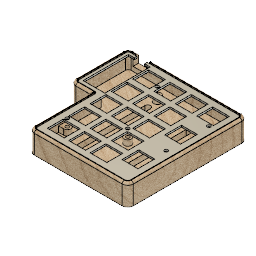
yampad_v3-Fusion360 (Autodesk Fusion 360 design; units mm, degrees)
Autodesk Fusion 360 part; units mm, degrees
note: some values were not read from the file. Set by a fixed rule: which sketch regions a step uses.
(part 1 of 2)
sketch "yampad_v2-Eco2.User-screws" plane through (0, 0, 0) normal (0, 1, 0) x (1, 0, 0) in component "Plate"
  line L0 (16.764, -31.877) -> (-1.397, -31.877) construction
  line L1 (71.501, -52.959) -> (57.531, -52.959) construction
  circle A0 centre (20.066, -74.613) radius 3.2553 construction
  line L2 (76.581, -81.534) -> (76.581, -67.564) construction
  line L3 (38.481, -0.889) -> (52.451, -0.889) construction
  line L4 (57.531, -52.959) -> (57.531, -38.989) construction
  line L5 (52.451, -0.889) -> (52.451, -14.859) construction
  line L6 (90.551, -67.564) -> (90.551, -81.534) construction
  circle A1 centre (54.991, -55.499) radius 3.2528 construction
  line L7 (33.401, -0.889) -> (33.401, -14.859) construction
  line L8 (90.551, -81.534) -> (76.581, -81.534) construction
  line L9 (11.557, -2.286) -> (3.937, -2.286) construction
  line L10 (3.937, 3.048) -> (11.557, 3.048) construction
  line L11 (3.937, -2.286) -> (3.937, 3.048) construction
  line L12 (57.531, -38.989) -> (71.501, -38.989) construction
  line L13 (16.764, 1.524) -> (16.764, -31.877) construction
  line L14 (33.401, -14.859) -> (19.431, -14.859) construction
  line L15 (19.431, -0.889) -> (33.401, -0.889) construction
  line L16 (-1.397, 1.524) -> (16.764, 1.524) construction
  line L17 (19.431, -14.859) -> (19.431, -0.889) construction
  line L18 (76.581, -29.464) -> (90.551, -29.464) construction
  line L19 (11.557, 3.048) -> (11.557, -2.286) construction
  line L20 (90.551, -43.434) -> (76.581, -43.434) construction
  line L21 (71.501, -38.989) -> (71.501, -52.959) construction
  line L22 (-1.397, -31.877) -> (-1.524, 1.524) construction
  line L23 (33.401, -33.909) -> (19.431, -33.909) construction
  line L24 (52.451, -14.859) -> (38.481, -14.859) construction
  line L25 (38.481, -52.959) -> (38.481, -38.989) construction
  line L26 (38.481, -33.909) -> (38.481, -19.939) construction
  line L27 (33.401, -58.039) -> (33.401, -72.009) construction
  line L28 (33.401, -19.939) -> (33.401, -33.909) construction
  line L29 (57.531, -58.039) -> (71.501, -58.039) construction
  line L30 (90.551, -14.859) -> (76.581, -14.859) construction
  line L31 (76.581, -43.434) -> (76.581, -29.464) construction
  line L32 (71.501, -33.909) -> (57.531, -33.909) construction
  line L33 (52.451, -52.959) -> (38.481, -52.959) construction
  line L34 (57.531, -33.909) -> (57.531, -19.939) construction
  line L35 (33.401, -52.959) -> (19.431, -52.959) construction
  line L36 (19.431, -52.959) -> (19.431, -38.989) construction
  line L37 (19.431, -19.939) -> (33.401, -19.939) construction
  line L38 (71.501, -19.939) -> (71.501, -33.909) construction
  line L39 (57.531, -14.859) -> (57.531, -0.889) construction
  line L40 (38.481, -14.859) -> (38.481, -0.889) construction
  circle A2 centre (35.941, -9.906) radius 3.2553 construction
  circle A3 centre (89.408, -17.399) radius 3.2453 construction
  line L41 (38.481, -19.939) -> (52.451, -19.939) construction
  line L42 (57.531, -19.939) -> (71.501, -19.939) construction
  line L43 (57.531, -0.889) -> (71.501, -0.889) construction
  line L44 (71.501, -14.859) -> (57.531, -14.859) construction
  line L45 (76.581, -14.859) -> (76.581, -0.889) construction
  line L46 (52.451, -19.939) -> (52.451, -33.909) construction
  line L47 (33.401, -38.989) -> (33.401, -52.959) construction
  line L48 (76.581, -67.564) -> (90.551, -67.564) construction
  circle A4 centre (89.408, -55.499) radius 3.2379 construction
  line L49 (52.451, -33.909) -> (38.481, -33.909) construction
  line L50 (90.551, -0.889) -> (90.551, -14.859) construction
  line L51 (19.431, -58.039) -> (33.401, -58.039) construction
  line L52 (76.581, -0.889) -> (90.551, -0.889) construction
  line L53 (38.481, -72.009) -> (38.481, -58.039) construction
  line L54 (38.481, -38.989) -> (52.451, -38.989) construction
  line L55 (19.431, -38.989) -> (33.401, -38.989) construction
  line L56 (33.401, -77.089) -> (33.401, -91.059) construction
  line L57 (71.501, -58.039) -> (71.501, -72.009) construction
  line L58 (52.451, -91.059) -> (38.481, -91.059) construction
  line L59 (19.431, -72.009) -> (19.431, -58.039) construction
  line L60 (90.551, -29.464) -> (90.551, -43.434) construction
  line L61 (52.451, -38.989) -> (52.451, -52.959) construction
  line L62 (71.501, -0.889) -> (71.501, -14.859) construction
  line L63 (19.431, -33.909) -> (19.431, -19.939) construction
  line L64 (71.501, -91.059) -> (57.531, -91.059) construction
  line L65 (33.401, -72.009) -> (19.431, -72.009) construction
  line L66 (57.531, -72.009) -> (57.531, -58.039) construction
  line L67 (38.481, -91.059) -> (38.481, -77.089) construction
  line L68 (19.431, -91.059) -> (19.431, -77.089) construction
  line L69 (52.451, -77.089) -> (52.451, -91.059) construction
  line L70 (57.531, -77.089) -> (71.501, -77.089) construction
  line L71 (71.501, -77.089) -> (71.501, -91.059) construction
  line L72 (52.451, -72.009) -> (38.481, -72.009) construction
  line L73 (71.501, -72.009) -> (57.531, -72.009) construction
  line L74 (19.431, -77.089) -> (33.401, -77.089) construction
  line L75 (38.481, -58.039) -> (52.451, -58.039) construction
  line L76 (52.451, -58.039) -> (52.451, -72.009) construction
  line L77 (33.401, -91.059) -> (19.431, -91.059) construction
  line L78 (57.531, -91.059) -> (57.531, -77.089) construction
  line L79 (38.481, -77.089) -> (52.451, -77.089) construction
sketch "yampad_v2-Edge.Cuts" plane through (0, 0, 0) normal (0, 1, 0) x (1, 0, 0) in component "Plate"
  arc A0 (16.51, -91.694) -> (18.288, -93.472) centre (18.288, -91.694) ccw construction
  line L0 (18.288, -93.472) -> (91.44, -93.472) construction
  line L1 (15.24, -38.354) -> (-0.254, -38.354) construction
  arc A1 (-1.524, -37.084) -> (-0.254, -38.354) centre (-0.254, -37.084) ccw construction
  line L2 (-1.524, -37.084) -> (-1.524, 0) construction
  line L3 (91.186, 1.524) -> (0, 1.524) construction
  arc A2 (0, 1.524) -> (-1.524, 0) centre (0, 0) ccw construction
  arc A3 (92.964, -0.254) -> (91.186, 1.524) centre (91.186, -0.254) ccw construction
  line L4 (16.51, -91.694) -> (16.51, -39.624) construction
  arc A4 (16.51, -39.624) -> (15.24, -38.354) centre (15.24, -39.624) ccw construction
  line L5 (92.964, -91.948) -> (92.964, -0.254) construction
  arc A5 (91.44, -93.472) -> (92.964, -91.948) centre (91.44, -91.948) ccw construction
sketch "Sketch3" plane through (0, 0, 0) normal (0, 1, 0) x (1, 0, 0) in component "Plate"
  line L0 (18.288, -93.472) -> (91.44, -93.472) construction
  arc A0 (16.51, -91.694) -> (18.288, -93.472) centre (18.288, -91.694) ccw construction
  line L1 (16.51, -91.694) -> (16.51, -39.624) construction
  arc A1 (16.51, -39.624) -> (15.24, -38.354) centre (15.24, -39.624) ccw construction
  line L2 (15.24, -38.354) -> (-0.254, -38.354) construction
  arc A2 (-1.524, -37.084) -> (-0.254, -38.354) centre (-0.254, -37.084) ccw construction
  line L3 (-1.524, -37.084) -> (-1.524, 0) construction
  arc A3 (0, 1.524) -> (-1.524, 0) centre (0, 0) ccw construction
  line L4 (91.186, 1.524) -> (0, 1.524) construction
  arc A4 (92.964, -0.254) -> (91.186, 1.524) centre (91.186, -0.254) ccw construction
  line L5 (92.964, -91.948) -> (92.964, -0.254) construction
  arc A5 (91.44, -93.472) -> (92.964, -91.948) centre (91.44, -91.948) ccw construction
  line L6 (91.44, -93.472) -> (92.964, -93.472) construction
  line L7 (92.964, -93.472) -> (92.964, -91.948) construction
  line L8 (91.186, 1.524) -> (92.964, 1.524) construction
  line L9 (92.964, 1.524) -> (92.964, -0.254) construction
  line L10 (-1.524, 0) -> (-1.524, 1.524) construction
  line L11 (0, 1.524) -> (-1.524, 1.524) construction
  line L12 (-1.524, -37.084) -> (-1.524, -38.354) construction
  line L13 (-1.524, -38.354) -> (-0.254, -38.354) construction
  line L14 (16.51, -91.694) -> (16.51, -93.472) construction
  line L15 (16.51, -93.472) -> (18.288, -93.472) construction
  line L16 (18.288, -96.472) -> (91.44, -96.472)
  line L17 (91.44, -96.472) -> (93.964, -96.472)
  line L18 (95.964, -94.472) -> (95.964, -91.948)
  line L19 (95.964, -91.948) -> (95.964, -0.254)
  line L20 (95.964, 2.524) -> (95.964, -0.254)
  line L21 (91.186, 4.524) -> (93.964, 4.524)
  line L22 (91.186, 4.524) -> (0, 4.524)
  line L23 (0, 4.524) -> (-2.524, 4.524)
  line L24 (-4.524, 0) -> (-4.524, 2.524)
  line L25 (-4.524, -37.084) -> (-4.524, 0)
  line L26 (-4.524, -37.084) -> (-4.524, -39.354)
  line L27 (-2.524, -41.354) -> (-0.254, -41.354)
  line L28 (11.51, -41.354) -> (-0.254, -41.354)
  line L29 (13.51, -91.694) -> (13.51, -43.354)
  line L30 (13.51, -91.694) -> (13.51, -94.472)
  line L31 (15.51, -96.472) -> (18.288, -96.472)
  arc A6 (95.964, 2.524) -> (93.964, 4.524) centre (93.964, 2.524) ccw
  arc A7 (-2.524, 4.524) -> (-4.524, 2.524) centre (-2.524, 2.524) ccw
  arc A8 (-4.524, -39.354) -> (-2.524, -41.354) centre (-2.524, -39.354) ccw
  arc A9 (13.51, -43.354) -> (11.51, -41.354) centre (11.51, -43.354) ccw
  arc A10 (13.51, -94.472) -> (15.51, -96.472) centre (15.51, -94.472) ccw
  arc A11 (93.964, -96.472) -> (95.964, -94.472) centre (93.964, -94.472) ccw
  point P0 (16.51, -91.694)
  point P1 (18.288, -93.472)
  dimension "d5" = 2
  dimension "d6" = 2
  dimension "d7" = 2
  dimension "d8" = 2
  constraint coincident L0.end A5.start
  constraint tangent A5 L6
  constraint coincident L5.start A5.end
  constraint tangent A5 L7
  constraint coincident L4.start A4.end
  constraint tangent A4 L8
  constraint coincident A4.start L5.end
  constraint tangent A4 L9
  constraint coincident L3.end A3.end
  constraint tangent A3 L10
  constraint coincident A3.start L4.end
  constraint tangent A3 L11
  constraint coincident A2.start L3.start
  constraint tangent A2 L12
  constraint coincident L2.end A2.end
  constraint tangent A2 L13
  constraint coincident P0 A0.start
  constraint tangent A0 L14
  constraint coincident P1 L0.start
  constraint tangent A0 L15
  constraint parallel L0 L16
  constraint parallel L6 L17
  constraint parallel L7 L18
  constraint parallel L5 L19
  constraint parallel L9 L20
  constraint parallel L8 L21
  constraint parallel L4 L22
  constraint parallel L11 L23
  constraint parallel L10 L24
  constraint parallel L3 L25
  constraint parallel L12 L26
  constraint parallel L13 L27
  constraint parallel L2 L28
  constraint parallel L1 L29
  constraint parallel L14 L30
  constraint parallel L15 L31
  constraint tangent L20 A6
  constraint tangent L21 A6
  constraint tangent L23 A7
  constraint tangent L24 A7
  constraint tangent L26 A8
  constraint tangent L27 A8
  constraint equal A7 A8
  constraint tangent L28 A9
  constraint tangent L29 A9
  constraint tangent L30 A10
  constraint tangent L31 A10
  constraint equal A9 A10
  constraint tangent L17 A11
  constraint tangent L18 A11
  measures "d5" radius of A6
  measures "d6" radius of A7
  measures "d7" radius of A9
  measures "d8" radius of A11
extrude "Extrude1" add sketch "Sketch3" along normal blind 1.5 makes body 1 in component "Plate"
sketch "Sketch4" plane through (0, 1.5, 0) normal (0, 1, 0) x (-1, 0, 0) in component "Plate"
  line L0 (-13.51, 43.354) -> (-13.51, 94.472)
  arc A0 (-13.51, 94.472) -> (-15.51, 96.472) centre (-15.51, 94.472) ccw
  line L1 (-15.51, 96.472) -> (-93.964, 96.472)
  arc A1 (-93.964, 96.472) -> (-95.964, 94.472) centre (-93.964, 94.472) ccw
  line L2 (-95.964, 94.472) -> (-95.964, -2.524)
  arc A2 (-95.964, -2.524) -> (-93.964, -4.524) centre (-93.964, -2.524) ccw
  line L3 (-93.964, -4.524) -> (2.524, -4.524)
  arc A3 (2.524, -4.524) -> (4.524, -2.524) centre (2.524, -2.524) ccw
  line L4 (4.524, -2.524) -> (4.524, 39.354)
  arc A4 (4.524, 39.354) -> (2.524, 41.354) centre (2.524, 39.354) ccw
  line L5 (2.524, 41.354) -> (-11.51, 41.354)
  arc A5 (-13.51, 43.354) -> (-11.51, 41.354) centre (-11.51, 43.354) ccw
  line L6 (-90.551, 29.464) -> (-90.551, 43.434) construction
  line L7 (1.397, 31.877) -> (1.524, -1.524) construction
  line L8 (-16.764, -1.524) -> (-16.764, 31.877) construction
  line L9 (-16.764, 31.877) -> (1.397, 31.877) construction
  line L10 (-3.937, 2.286) -> (-3.937, -3.048) construction
  line L11 (-3.937, -3.048) -> (-11.557, -3.048) construction
  line L12 (-11.557, -3.048) -> (-11.557, 2.286) construction
  line L13 (-11.557, 2.286) -> (-3.937, 2.286) construction
  line L14 (1.397, -1.524) -> (-16.764, -1.524) construction
  line L15 (-19.431, 0.889) -> (-33.401, 0.889) construction
  line L16 (-19.431, 14.859) -> (-19.431, 0.889) construction
  line L17 (-33.401, 14.859) -> (-19.431, 14.859) construction
  line L18 (-33.401, 0.889) -> (-33.401, 14.859) construction
  circle A6 centre (-35.941, 9.906) radius 3.2553 construction
  line L19 (-38.481, 14.859) -> (-38.481, 0.889) construction
  line L20 (-38.481, 0.889) -> (-52.451, 0.889) construction
  line L21 (-52.451, 0.889) -> (-52.451, 14.859) construction
  line L22 (-52.451, 14.859) -> (-38.481, 14.859) construction
  line L23 (-57.531, 14.859) -> (-57.531, 0.889) construction
  line L24 (-57.531, 0.889) -> (-71.501, 0.889) construction
  line L25 (-71.501, 0.889) -> (-71.501, 14.859) construction
  line L26 (-71.501, 14.859) -> (-57.531, 14.859) construction
  line L27 (-76.581, 14.859) -> (-76.581, 0.889) construction
  line L28 (-76.581, 0.889) -> (-90.551, 0.889) construction
  line L29 (-90.551, 0.889) -> (-90.551, 14.859) construction
  line L30 (-90.551, 14.859) -> (-76.581, 14.859) construction
  circle A7 centre (-89.408, 17.399) radius 3.2453 construction
  line L31 (-76.581, 29.464) -> (-90.551, 29.464) construction
  line L32 (-76.581, 43.434) -> (-76.581, 29.464) construction
  line L33 (-90.551, 43.434) -> (-76.581, 43.434) construction
  circle A8 centre (-89.408, 55.499) radius 3.2379 construction
  line L34 (-76.581, 67.564) -> (-90.551, 67.564) construction
  line L35 (-90.551, 67.564) -> (-90.551, 81.534) construction
  line L36 (-90.551, 81.534) -> (-76.581, 81.534) construction
  line L37 (-76.581, 81.534) -> (-76.581, 67.564) construction
  line L38 (-71.501, 77.089) -> (-71.501, 91.059) construction
  line L39 (-57.531, 77.089) -> (-71.501, 77.089) construction
  line L40 (-57.531, 91.059) -> (-57.531, 77.089) construction
  line L41 (-71.501, 91.059) -> (-57.531, 91.059) construction
  line L42 (-52.451, 91.059) -> (-38.481, 91.059) construction
  line L43 (-52.451, 77.089) -> (-52.451, 91.059) construction
  line L44 (-38.481, 77.089) -> (-52.451, 77.089) construction
  line L45 (-38.481, 91.059) -> (-38.481, 77.089) construction
  line L46 (-33.401, 91.059) -> (-19.431, 91.059) construction
  line L47 (-19.431, 91.059) -> (-19.431, 77.089) construction
  line L48 (-19.431, 77.089) -> (-33.401, 77.089) construction
  line L49 (-33.401, 77.089) -> (-33.401, 91.059) construction
  circle A9 centre (-20.066, 74.613) radius 3.2553 construction
  line L50 (-19.431, 58.039) -> (-33.401, 58.039) construction
  line L51 (-33.401, 58.039) -> (-33.401, 72.009) construction
  line L52 (-19.431, 72.009) -> (-19.431, 58.039) construction
  line L53 (-33.401, 72.009) -> (-19.431, 72.009) construction
  line L54 (-38.481, 58.039) -> (-52.451, 58.039) construction
  line L55 (-52.451, 58.039) -> (-52.451, 72.009) construction
  line L56 (-38.481, 72.009) -> (-38.481, 58.039) construction
  line L57 (-52.451, 72.009) -> (-38.481, 72.009) construction
  line L58 (-57.531, 58.039) -> (-71.501, 58.039) construction
  line L59 (-71.501, 58.039) -> (-71.501, 72.009) construction
  line L60 (-57.531, 72.009) -> (-57.531, 58.039) construction
  line L61 (-71.501, 72.009) -> (-57.531, 72.009) construction
  line L62 (-57.531, 38.989) -> (-71.501, 38.989) construction
  line L63 (-71.501, 38.989) -> (-71.501, 52.959) construction
  line L64 (-57.531, 52.959) -> (-57.531, 38.989) construction
  line L65 (-71.501, 52.959) -> (-57.531, 52.959) construction
  line L66 (-38.481, 38.989) -> (-52.451, 38.989) construction
  line L67 (-52.451, 38.989) -> (-52.451, 52.959) construction
  line L68 (-38.481, 52.959) -> (-38.481, 38.989) construction
  line L69 (-52.451, 52.959) -> (-38.481, 52.959) construction
  line L70 (-19.431, 38.989) -> (-33.401, 38.989) construction
  line L71 (-33.401, 38.989) -> (-33.401, 52.959) construction
  line L72 (-19.431, 52.959) -> (-19.431, 38.989) construction
  line L73 (-33.401, 52.959) -> (-19.431, 52.959) construction
  line L74 (-19.431, 19.939) -> (-33.401, 19.939) construction
  line L75 (-33.401, 19.939) -> (-33.401, 33.909) construction
  line L76 (-19.431, 33.909) -> (-19.431, 19.939) construction
  line L77 (-33.401, 33.909) -> (-19.431, 33.909) construction
  line L78 (-38.481, 19.939) -> (-52.451, 19.939) construction
  line L79 (-52.451, 19.939) -> (-52.451, 33.909) construction
  line L80 (-38.481, 33.909) -> (-38.481, 19.939) construction
  line L81 (-52.451, 33.909) -> (-38.481, 33.909) construction
  line L82 (-57.531, 19.939) -> (-71.501, 19.939) construction
  line L83 (-71.501, 19.939) -> (-71.501, 33.909) construction
  line L84 (-57.531, 33.909) -> (-57.531, 19.939) construction
  line L85 (-71.501, 33.909) -> (-57.531, 33.909) construction
  circle A10 centre (-54.991, 55.499) radius 3.2528 construction
  circle A11 centre (-35.941, 9.906) radius 1.5875
  circle A12 centre (-89.408, 17.399) radius 1.5875
  circle A13 centre (-89.408, 55.499) radius 1.5875
  circle A14 centre (-54.991, 55.499) radius 1.5875
  circle A15 centre (-20.066, 74.613) radius 1.5875
  line L86 (-3.937, -3.048) -> (-11.557, 2.286) construction
  line L87 (-12.247, -4.524) -> (-3.247, -4.524)
  line L88 (-3.247, -4.524) -> (-3.247, 3.762)
  line L89 (-3.247, 3.762) -> (-12.247, 3.762)
  line L90 (-12.247, 3.762) -> (-12.247, -4.524)
  line L91 (-12.247, -4.524) -> (-3.247, 3.762) construction
  line L92 (-3.247, -4.524) -> (-12.247, 3.762) construction
  line L93 (-19.431, 0.889) -> (-33.401, 14.859) construction
  line L94 (-38.481, 0.889) -> (-52.451, 14.859) construction
  line L95 (-57.531, 0.889) -> (-71.501, 14.859) construction
  line L96 (-76.581, 0.889) -> (-90.551, 14.859) construction
  line L97 (-19.431, 19.939) -> (-33.401, 33.909) construction
  line L98 (-19.431, 38.989) -> (-33.401, 52.959) construction
  line L99 (-38.481, 38.989) -> (-52.451, 52.959) construction
  line L100 (-38.481, 19.939) -> (-52.451, 33.909) construction
  line L101 (-57.531, 19.939) -> (-71.501, 33.909) construction
  line L102 (-57.531, 38.989) -> (-71.501, 52.959) construction
  line L103 (-76.581, 29.464) -> (-90.551, 43.434) construction
  line L104 (-19.431, 58.039) -> (-33.401, 72.009) construction
  line L105 (-38.481, 58.039) -> (-52.451, 72.009) construction
  line L106 (-57.531, 58.039) -> (-71.501, 72.009) construction
  line L107 (-76.581, 67.564) -> (-90.551, 81.534) construction
  line L108 (-19.431, 77.089) -> (-33.401, 91.059) construction
  line L109 (-38.481, 77.089) -> (-52.451, 91.059) construction
  line L110 (-57.531, 77.089) -> (-71.501, 91.059) construction
  line L111 (-33.916, 14.974) -> (-18.916, 14.974)
  line L112 (-18.916, 14.974) -> (-18.916, 0.774)
  line L113 (-18.916, 0.774) -> (-33.916, 0.774)
  line L114 (-33.916, 0.774) -> (-33.916, 14.974)
  line L115 (-33.916, 14.974) -> (-18.916, 0.774) construction
  line L116 (-18.916, 14.974) -> (-33.916, 0.774) construction
  line L117 (-37.966, 14.974) -> (-52.966, 14.974)
  line L118 (-52.966, 14.974) -> (-52.966, 0.774)
  line L119 (-52.966, 0.774) -> (-37.966, 0.774)
  line L120 (-37.966, 0.774) -> (-37.966, 14.974)
  line L121 (-37.966, 14.974) -> (-52.966, 0.774) construction
  line L122 (-52.966, 14.974) -> (-37.966, 0.774) construction
  line L123 (-72.016, 14.974) -> (-57.016, 14.974)
  line L124 (-57.016, 14.974) -> (-57.016, 0.774)
  line L125 (-57.016, 0.774) -> (-72.016, 0.774)
  line L126 (-72.016, 0.774) -> (-72.016, 14.974)
  line L127 (-72.016, 14.974) -> (-57.016, 0.774) construction
  line L128 (-57.016, 14.974) -> (-72.016, 0.774) construction
  line L129 (-91.066, 14.974) -> (-76.066, 14.974)
  line L130 (-76.066, 14.974) -> (-76.066, 0.774)
  line L131 (-76.066, 0.774) -> (-91.066, 0.774)
  line L132 (-91.066, 0.774) -> (-91.066, 14.974)
  line L133 (-91.066, 14.974) -> (-76.066, 0.774) construction
  line L134 (-76.066, 14.974) -> (-91.066, 0.774) construction
  line L135 (-33.916, 34.024) -> (-18.916, 34.024)
  line L136 (-18.916, 34.024) -> (-18.916, 19.824)
  line L137 (-18.916, 19.824) -> (-33.916, 19.824)
  line L138 (-33.916, 19.824) -> (-33.916, 34.024)
  line L139 (-33.916, 34.024) -> (-18.916, 19.824) construction
  line L140 (-18.916, 34.024) -> (-33.916, 19.824) construction
  line L141 (-52.966, 19.824) -> (-37.966, 19.824)
  line L142 (-37.966, 19.824) -> (-37.966, 34.024)
  line L143 (-37.966, 34.024) -> (-52.966, 34.024)
  line L144 (-52.966, 34.024) -> (-52.966, 19.824)
  line L145 (-52.966, 19.824) -> (-37.966, 34.024) construction
  line L146 (-37.966, 19.824) -> (-52.966, 34.024) construction
  line L147 (-72.016, 34.024) -> (-57.016, 34.024)
  line L148 (-57.016, 34.024) -> (-57.016, 19.824)
  line L149 (-57.016, 19.824) -> (-72.016, 19.824)
  line L150 (-72.016, 19.824) -> (-72.016, 34.024)
  line L151 (-72.016, 34.024) -> (-57.016, 19.824) construction
  line L152 (-57.016, 34.024) -> (-72.016, 19.824) construction
  line L153 (-90.666, 43.949) -> (-76.466, 43.949)
  line L154 (-76.466, 43.949) -> (-76.466, 28.949)
  line L155 (-76.466, 28.949) -> (-90.666, 28.949)
  line L156 (-90.666, 28.949) -> (-90.666, 43.949)
  line L157 (-90.666, 43.949) -> (-76.466, 28.949) construction
  line L158 (-76.466, 43.949) -> (-90.666, 28.949) construction
  line L159 (-33.916, 53.074) -> (-18.916, 53.074)
  line L160 (-18.916, 53.074) -> (-18.916, 38.874)
  line L161 (-18.916, 38.874) -> (-33.916, 38.874)
  line L162 (-33.916, 38.874) -> (-33.916, 53.074)
  line L163 (-33.916, 53.074) -> (-18.916, 38.874) construction
  line L164 (-18.916, 53.074) -> (-33.916, 38.874) construction
  line L165 (-52.966, 53.074) -> (-37.966, 53.074)
  line L166 (-37.966, 53.074) -> (-37.966, 38.874)
  line L167 (-37.966, 38.874) -> (-52.966, 38.874)
  line L168 (-52.966, 38.874) -> (-52.966, 53.074)
  line L169 (-52.966, 53.074) -> (-37.966, 38.874) construction
  line L170 (-37.966, 53.074) -> (-52.966, 38.874) construction
  line L171 (-72.016, 53.074) -> (-57.016, 53.074)
  line L172 (-57.016, 53.074) -> (-57.016, 38.874)
  line L173 (-57.016, 38.874) -> (-72.016, 38.874)
  line L174 (-72.016, 38.874) -> (-72.016, 53.074)
  line L175 (-72.016, 53.074) -> (-57.016, 38.874) construction
  line L176 (-57.016, 53.074) -> (-72.016, 38.874) construction
  line L177 (-33.916, 72.124) -> (-18.916, 72.124)
  line L178 (-18.916, 72.124) -> (-18.916, 57.924)
  line L179 (-18.916, 57.924) -> (-33.916, 57.924)
  line L180 (-33.916, 57.924) -> (-33.916, 72.124)
  line L181 (-33.916, 72.124) -> (-18.916, 57.924) construction
  line L182 (-18.916, 72.124) -> (-33.916, 57.924) construction
  line L183 (-52.966, 72.124) -> (-37.966, 72.124)
  line L184 (-37.966, 72.124) -> (-37.966, 57.924)
  line L185 (-37.966, 57.924) -> (-52.966, 57.924)
  line L186 (-52.966, 57.924) -> (-52.966, 72.124)
  line L187 (-52.966, 72.124) -> (-37.966, 57.924) construction
  line L188 (-37.966, 72.124) -> (-52.966, 57.924) construction
  line L189 (-72.016, 72.124) -> (-57.016, 72.124)
  line L190 (-57.016, 72.124) -> (-57.016, 57.924)
  line L191 (-57.016, 57.924) -> (-72.016, 57.924)
  line L192 (-72.016, 57.924) -> (-72.016, 72.124)
  line L193 (-72.016, 72.124) -> (-57.016, 57.924) construction
  line L194 (-57.016, 72.124) -> (-72.016, 57.924) construction
  line L195 (-90.666, 82.049) -> (-76.466, 82.049)
  line L196 (-76.466, 82.049) -> (-76.466, 67.049)
  line L197 (-76.466, 67.049) -> (-90.666, 67.049)
  line L198 (-90.666, 67.049) -> (-90.666, 82.049)
  line L199 (-90.666, 82.049) -> (-76.466, 67.049) construction
  line L200 (-76.466, 82.049) -> (-90.666, 67.049) construction
  line L201 (-33.916, 91.174) -> (-18.916, 91.174)
  line L202 (-18.916, 91.174) -> (-18.916, 76.974)
  line L203 (-18.916, 76.974) -> (-33.916, 76.974)
  line L204 (-33.916, 76.974) -> (-33.916, 91.174)
  line L205 (-33.916, 91.174) -> (-18.916, 76.974) construction
  line L206 (-18.916, 91.174) -> (-33.916, 76.974) construction
  line L207 (-52.966, 91.174) -> (-37.966, 91.174)
  line L208 (-37.966, 91.174) -> (-37.966, 76.974)
  line L209 (-37.966, 76.974) -> (-52.966, 76.974)
  line L210 (-52.966, 76.974) -> (-52.966, 91.174)
  line L211 (-52.966, 91.174) -> (-37.966, 76.974) construction
  line L212 (-37.966, 91.174) -> (-52.966, 76.974) construction
  line L213 (-72.016, 91.174) -> (-57.016, 91.174)
  line L214 (-57.016, 91.174) -> (-57.016, 76.974)
  line L215 (-57.016, 76.974) -> (-72.016, 76.974)
  line L216 (-72.016, 76.974) -> (-72.016, 91.174)
  line L217 (-72.016, 91.174) -> (-57.016, 76.974) construction
  line L218 (-57.016, 91.174) -> (-72.016, 76.974) construction
  line L219 (2.024, -2.524) -> (2.024, 39.354) construction
  line L220 (-15.24, 38.354) -> (0.254, 38.354)
  line L221 (1.397, -2.174) -> (-17.414, -2.174)
  line L222 (-17.414, -2.174) -> (-17.414, 32.527)
  line L223 (-17.414, 32.527) -> (1.397, 32.527) construction
  line L224 (1.397, 32.527) -> (2.024, 32.527)
  line L225 (2.024, 32.527) -> (2.024, -2.4)
  line L226 (1.397, -2.174) -> (2.0241, -2.174)
  line L227 (-17.414, 32.527) -> (-17.414, 38.354)
  line L228 (-17.414, 38.354) -> (2.024, 38.354)
  line L229 (2.024, 38.354) -> (2.024, 32.527)
  point P0 (-3.937, -3.048)
  point P1 (-7.747, -0.381)
  point P2 (-26.416, 7.874)
  point P3 (-45.466, 7.874)
  point P4 (-64.516, 7.874)
  point P5 (-83.566, 7.874)
  point P6 (-26.416, 26.924)
  point P7 (-45.466, 26.924)
  point P8 (-64.516, 26.924)
  point P9 (-83.566, 36.449)
  point P10 (-26.416, 45.974)
  point P11 (-45.466, 45.974)
  point P12 (-64.516, 45.974)
  point P13 (-26.416, 65.024)
  point P14 (-45.466, 65.024)
  point P15 (-64.516, 65.024)
  point P16 (-83.566, 74.549)
  point P17 (-26.416, 84.074)
  point P18 (-45.466, 84.074)
  point P19 (-64.516, 84.074)
  dimension "d13" = 3.175
  dimension "d14" = 3.175
  dimension "d15" = 3.175
  dimension "d16" = 3.175
  dimension "d17" = 3.175
  dimension "d20" = 9
  dimension "d23" = 15
  dimension "d24" = 14.2
  dimension "d25" = 15
  dimension "d26" = 14.2
  dimension "d27" = 15
  dimension "d28" = 14.2
  dimension "d29" = 15
  dimension "d30" = 14.2
  dimension "d31" = 15
  dimension "d32" = 14.2
  dimension "d33" = 15
  dimension "d34" = 14.2
  dimension "d35" = 15
  dimension "d36" = 14.2
  dimension "d37" = 14.2
  dimension "d38" = 15
  dimension "d39" = 15
  dimension "d40" = 14.2
  dimension "d41" = 15
  dimension "d42" = 14.2
  dimension "d43" = 15
  dimension "d44" = 14.2
  dimension "d45" = 15
  dimension "d46" = 14.2
  dimension "d47" = 15
  dimension "d48" = 14.2
  dimension "d49" = 15
  dimension "d50" = 14.2
  dimension "d51" = 14.2
  dimension "d52" = 15
  dimension "d53" = 15
  dimension "d54" = 14.2
  dimension "d55" = 15
  dimension "d56" = 14.2
  dimension "d57" = 15
  dimension "d58" = 14.2
  dimension "d82" = -2.5
  dimension "d83" = -0.65
  constraint concentric A6 A11
  constraint concentric A7 A12
  constraint concentric A8 A13
  constraint concentric A10 A14
  constraint concentric A9 A15
  constraint coincident P0 L10.end
  constraint coincident L12.end L13.start
  constraint perpendicular L87 L88
  constraint parallel L87 L89
  constraint parallel L88 L90
  constraint horizontal L87
  constraint coincident L91 P1
  constraint coincident L92 P1
  constraint midpoint L86 P1
  constraint coincident L15.start L16.end
  constraint coincident L17.start L18.end
  constraint coincident L19.end L20.start
  constraint coincident L21.end L22.start
  constraint coincident L23.end L24.start
  constraint coincident L25.end L26.start
  constraint coincident L27.end L28.start
  constraint coincident L29.end L30.start
  constraint coincident L74.start L76.end
  constraint coincident L75.end L77.start
  constraint coincident L70.start L72.end
  constraint coincident L71.end L73.start
  constraint coincident L66.start L68.end
  constraint coincident L67.end L69.start
  constraint coincident L78.start L80.end
  constraint coincident L79.end L81.start
  constraint coincident L82.start L84.end
  constraint coincident L83.end L85.start
  constraint coincident L62.start L64.end
  constraint coincident L63.end L65.start
  constraint coincident L31.start L32.end
  constraint coincident L6.end L33.start
  constraint coincident L50.start L52.end
  constraint coincident L51.end L53.start
  constraint coincident L54.start L56.end
  constraint coincident L55.end L57.start
  constraint coincident L58.start L60.end
  constraint coincident L59.end L61.start
  constraint coincident L34.start L37.end
  constraint coincident L35.end L36.start
  constraint coincident L47.end L48.start
  constraint coincident L46.start L49.end
  constraint coincident L44.start L45.end
  constraint coincident L42.start L43.end
  constraint coincident L39.start L40.end
  constraint coincident L38.end L41.start
  constraint perpendicular L111 L112
  constraint parallel L111 L113
  constraint parallel L112 L114
  constraint horizontal L111
  constraint coincident L115 P2
  constraint coincident L116 P2
  constraint midpoint L93 P2
  constraint perpendicular L117 L118
  constraint parallel L117 L119
  constraint parallel L118 L120
  constraint horizontal L117
  constraint coincident L121 P3
  constraint coincident L122 P3
  constraint midpoint L94 P3
  constraint perpendicular L123 L124
  constraint parallel L123 L125
  constraint parallel L124 L126
  constraint horizontal L123
  constraint coincident L127 P4
  constraint coincident L128 P4
  constraint midpoint L95 P4
  constraint perpendicular L129 L130
  constraint parallel L129 L131
  constraint parallel L130 L132
  constraint horizontal L129
  constraint coincident L133 P5
  constraint coincident L134 P5
  constraint midpoint L96 P5
  constraint perpendicular L135 L136
  constraint parallel L135 L137
  constraint parallel L136 L138
  constraint horizontal L135
  constraint coincident L139 P6
  constraint coincident L140 P6
  constraint midpoint L97 P6
  constraint perpendicular L141 L142
  constraint parallel L141 L143
  constraint parallel L142 L144
  constraint horizontal L141
  constraint coincident L145 P7
  constraint coincident L146 P7
  constraint midpoint L100 P7
  constraint perpendicular L147 L148
  constraint parallel L147 L149
  constraint parallel L148 L150
  constraint horizontal L147
  constraint coincident L151 P8
  constraint coincident L152 P8
  constraint midpoint L101 P8
  constraint perpendicular L153 L154
  constraint parallel L153 L155
  constraint parallel L154 L156
  constraint horizontal L153
  constraint coincident L157 P9
  constraint coincident L158 P9
  constraint midpoint L103 P9
  constraint perpendicular L159 L160
  constraint parallel L159 L161
  constraint parallel L160 L162
  constraint horizontal L159
  constraint coincident L163 P10
  constraint coincident L164 P10
  constraint midpoint L98 P10
  constraint perpendicular L165 L166
  constraint parallel L165 L167
  constraint parallel L166 L168
  constraint horizontal L165
  constraint coincident L169 P11
  constraint coincident L170 P11
  constraint midpoint L99 P11
  constraint perpendicular L171 L172
  constraint parallel L171 L173
  constraint parallel L172 L174
  constraint horizontal L171
  constraint coincident L175 P12
  constraint coincident L176 P12
  constraint midpoint L102 P12
  constraint perpendicular L177 L178
  constraint parallel L177 L179
  constraint parallel L178 L180
  constraint horizontal L177
  constraint coincident L181 P13
  constraint coincident L182 P13
  constraint midpoint L104 P13
  constraint perpendicular L183 L184
  constraint parallel L183 L185
  constraint parallel L184 L186
  constraint horizontal L183
  constraint coincident L187 P14
  constraint coincident L188 P14
  constraint midpoint L105 P14
  constraint perpendicular L189 L190
  constraint parallel L189 L191
  constraint parallel L190 L192
  constraint horizontal L189
  constraint coincident L193 P15
  constraint coincident L194 P15
  constraint midpoint L106 P15
  constraint perpendicular L195 L196
  constraint parallel L195 L197
  constraint parallel L196 L198
  constraint horizontal L195
  constraint coincident L199 P16
  constraint coincident L200 P16
  constraint midpoint L107 P16
  constraint perpendicular L201 L202
  constraint parallel L201 L203
  constraint parallel L202 L204
  constraint horizontal L201
  constraint coincident L205 P17
  constraint coincident L206 P17
  constraint midpoint L108 P17
  constraint perpendicular L207 L208
  constraint parallel L207 L209
  constraint parallel L208 L210
  constraint horizontal L207
  constraint coincident L211 P18
  constraint coincident L212 P18
  constraint midpoint L109 P18
  constraint perpendicular L213 L214
  constraint parallel L213 L215
  constraint parallel L214 L216
  constraint horizontal L213
  constraint coincident L217 P19
  constraint coincident L218 P19
  constraint midpoint L110 P19
  constraint coincident L219 L224.end
  constraint perpendicular L219 L224
  constraint coincident L219 L225.end
  constraint perpendicular L221 L225
  constraint horizontal L226
  constraint perpendicular L223 L227
  constraint coincident L219 L228.end
  constraint perpendicular L219 L228
  measures "d13" diameter of A11
  measures "d14" diameter of A12
  measures "d15" diameter of A13
  measures "d16" diameter of A14
  measures "d17" diameter of A15
  measures "d20" distance of L88.end L89.end
  measures "d23" distance of L112.end L113.end
  measures "d24" distance of L111.end L112.end
  measures "d25" distance of L118.end L119.end
  measures "d26" distance of L117.end L118.end
  measures "d27" distance of L124.end L125.end
  measures "d28" distance of L123.end L124.end
  measures "d29" distance of L130.end L131.end
  measures "d30" distance of L129.end L130.end
  measures "d31" distance of L136.end L137.end
  measures "d32" distance of L135.end L136.end
  measures "d33" distance of L142.end L143.end
  measures "d34" distance of L141.end L142.end
  measures "d35" distance of L148.end L149.end
  measures "d36" distance of L147.end L148.end
  measures "d37" distance of L154.end L155.end
  measures "d38" distance of L153.end L154.end
  measures "d39" distance of L160.end L161.end
  measures "d40" distance of L159.end L160.end
  measures "d41" distance of L166.end L167.end
  measures "d42" distance of L165.end L166.end
  measures "d43" distance of L172.end L173.end
  measures "d44" distance of L171.end L172.end
  measures "d45" distance of L178.end L179.end
  measures "d46" distance of L177.end L178.end
  measures "d47" distance of L184.end L185.end
  measures "d48" distance of L183.end L184.end
  measures "d49" distance of L190.end L191.end
  measures "d50" distance of L189.end L190.end
  measures "d51" distance of L196.end L197.end
  measures "d52" distance of L195.end L196.end
  measures "d53" distance of L202.end L203.end
  measures "d54" distance of L201.end L202.end
  measures "d55" distance of L208.end L209.end
  measures "d56" distance of L207.end L208.end
  measures "d57" distance of L214.end L215.end
  measures "d58" distance of L213.end L214.end
extrude "Extrude2" cut sketch "Sketch4" against normal through all contours L3 L87 L88 L90 L221 | L88 L89 L90 L221 | L88 L89 L90 L220 L221 L222 L225 L226 L227 L228 L229 | A11 | A12 | A13 | A14 | A15 | L111 L112 L113 L114 | L117 L118 L119 L120 | L123 L124 L125 L126 | L129 L130 L131 L132 | L135 L136 L137 L138 | L141 L142 L143 L144 | L147 L148 L149 L150 | L153 L154 L155 L156 | L159 L160 L161 L162 | L165 L166 L167 L168 | L171 L172 L173 L174 | L177 L178 L179 L180 | L183 L184 L185 L186 | L189 L190 L191 L192 | L195 L196 L197 L198 | L201 L202 L203 L204 | L207 L208 L209 L210 | L213 L214 L215 L216 bodies 1 in component "Plate"
sketch "Sketch1" plane through (0, 0, 0) normal (0, 1, 0) x (1, 0, 0) in component "Case"
  line L0 (11.51, -41.354) -> (-0.254, -41.354) construction
  line L1 (-2.524, -41.354) -> (-0.254, -41.354) construction
  arc A0 (-4.524, -39.354) -> (-2.524, -41.354) centre (-2.524, -39.354) ccw construction
  line L2 (-4.524, -37.084) -> (-4.524, -39.354) construction
  line L3 (-4.524, -37.084) -> (-4.524, 0) construction
  line L4 (-4.524, 0) -> (-4.524, 2.524) construction
  arc A1 (-2.524, 4.524) -> (-4.524, 2.524) centre (-2.524, 2.524) ccw construction
  line L5 (0, 4.524) -> (-2.524, 4.524) construction
  line L6 (91.186, 4.524) -> (0, 4.524) construction
  line L7 (91.186, 4.524) -> (93.964, 4.524) construction
  arc A2 (95.964, 2.524) -> (93.964, 4.524) centre (93.964, 2.524) ccw construction
  line L8 (95.964, 2.524) -> (95.964, -0.254) construction
  line L9 (95.964, -91.948) -> (95.964, -0.254) construction
  line L10 (95.964, -94.472) -> (95.964, -91.948) construction
  arc A3 (93.964, -96.472) -> (95.964, -94.472) centre (93.964, -94.472) ccw construction
  line L11 (91.44, -96.472) -> (93.964, -96.472) construction
  line L12 (18.288, -96.472) -> (91.44, -96.472) construction
  line L13 (15.51, -96.472) -> (18.288, -96.472) construction
  arc A4 (13.51, -94.472) -> (15.51, -96.472) centre (15.51, -94.472) ccw construction
  line L14 (13.51, -91.694) -> (13.51, -94.472) construction
  arc A5 (13.51, -43.354) -> (11.51, -41.354) centre (11.51, -43.354) ccw construction
  line L15 (13.51, -91.694) -> (13.51, -43.354) construction
  line L16 (15.24, -38.354) -> (-0.254, -38.354) construction
  arc A6 (-1.524, -37.084) -> (-0.254, -38.354) centre (-0.254, -37.084) ccw construction
  line L17 (-1.524, -37.084) -> (-1.524, 0) construction
  arc A7 (0, 1.524) -> (-1.524, 0) centre (0, 0) ccw construction
  line L18 (91.186, 1.524) -> (0, 1.524) construction
  arc A8 (92.964, -0.254) -> (91.186, 1.524) centre (91.186, -0.254) ccw construction
  line L19 (92.964, -91.948) -> (92.964, -0.254) construction
  arc A9 (91.44, -93.472) -> (92.964, -91.948) centre (91.44, -91.948) ccw construction
  line L20 (18.288, -93.472) -> (91.44, -93.472) construction
  arc A10 (16.51, -91.694) -> (18.288, -93.472) centre (18.288, -91.694) ccw construction
  arc A11 (16.51, -39.624) -> (15.24, -38.354) centre (15.24, -39.624) ccw construction
  line L21 (16.51, -91.694) -> (16.51, -39.624) construction
  line L22 (98.964, 2.524) -> (98.964, -0.254)
  line L23 (98.964, -91.948) -> (98.964, -0.254)
  line L24 (98.964, -94.472) -> (98.964, -91.948)
  arc A12 (93.964, -99.472) -> (98.964, -94.472) centre (93.964, -94.472) ccw
  line L25 (91.44, -99.472) -> (93.964, -99.472)
  line L26 (18.288, -99.472) -> (91.44, -99.472)
  line L27 (15.51, -99.472) -> (18.288, -99.472)
  arc A13 (10.51, -94.472) -> (15.51, -99.472) centre (15.51, -94.472) ccw
  line L28 (10.51, -91.694) -> (10.51, -94.472)
  line L29 (10.51, -91.694) -> (10.51, -44.354)
  line L30 (10.51, -44.354) -> (-0.254, -44.354)
  line L31 (-2.524, -44.354) -> (-0.254, -44.354)
  arc A14 (-7.524, -39.354) -> (-2.524, -44.354) centre (-2.524, -39.354) ccw
  line L32 (-7.524, -37.084) -> (-7.524, -39.354)
  line L33 (-7.524, -37.084) -> (-7.524, 0)
  line L34 (-7.524, 0) -> (-7.524, 2.524)
  arc A15 (-2.524, 7.524) -> (-7.524, 2.524) centre (-2.524, 2.524) ccw
  line L35 (0, 7.524) -> (-2.524, 7.524)
  line L36 (91.186, 7.524) -> (0, 7.524)
  line L37 (91.186, 7.524) -> (93.964, 7.524)
  arc A16 (98.964, 2.524) -> (93.964, 7.524) centre (93.964, 2.524) ccw
  point P0 (0, 4.524)
  dimension "d60" = -3
extrude "Extrude1'" add sketch "Sketch1" against normal blind 19 separate body makes body 2 in component "Case"
sketch "Sketch2" plane through (0, 0, 0) normal (0, 1, 0) x (-1, 0, 0) in component "Case"
  line L0 (-10.51, 44.354) -> (-10.51, 94.472) construction
  arc A0 (-10.51, 94.472) -> (-15.51, 99.472) centre (-15.51, 94.472) ccw construction
  line L1 (-15.51, 99.472) -> (-93.964, 99.472) construction
  arc A1 (-93.964, 99.472) -> (-98.964, 94.472) centre (-93.964, 94.472) ccw construction
  line L2 (-98.964, 94.472) -> (-98.964, -2.524) construction
  arc A2 (-98.964, -2.524) -> (-93.964, -7.524) centre (-93.964, -2.524) ccw construction
  line L3 (-93.964, -7.524) -> (2.524, -7.524) construction
  arc A3 (2.524, -7.524) -> (7.524, -2.524) centre (2.524, -2.524) ccw construction
  line L4 (7.524, -2.524) -> (7.524, 39.354) construction
  arc A4 (7.524, 39.354) -> (2.524, 44.354) centre (2.524, 39.354) ccw construction
  line L5 (2.524, 44.354) -> (-10.51, 44.354) construction
  line L6 (2.524, 41.354) -> (0.254, 41.354) construction
  arc A5 (4.524, 39.354) -> (2.524, 41.354) centre (2.524, 39.354) ccw construction
  line L7 (4.524, 37.084) -> (4.524, 39.354) construction
  line L8 (4.524, 37.084) -> (4.524, 0) construction
  line L9 (4.524, 0) -> (4.524, -2.524) construction
  arc A6 (2.524, -4.524) -> (4.524, -2.524) centre (2.524, -2.524) ccw construction
  line L10 (0, -4.524) -> (2.524, -4.524) construction
  line L11 (-91.186, -4.524) -> (0, -4.524) construction
  line L12 (-91.186, -4.524) -> (-93.964, -4.524) construction
  arc A7 (-95.964, -2.524) -> (-93.964, -4.524) centre (-93.964, -2.524) ccw construction
  line L13 (-95.964, -2.524) -> (-95.964, 0.254) construction
  line L14 (-95.964, 91.948) -> (-95.964, 0.254) construction
  line L15 (-95.964, 94.472) -> (-95.964, 91.948) construction
  arc A8 (-93.964, 96.472) -> (-95.964, 94.472) centre (-93.964, 94.472) ccw construction
  line L16 (-91.44, 96.472) -> (-93.964, 96.472) construction
  line L17 (-18.288, 96.472) -> (-91.44, 96.472) construction
  line L18 (-15.51, 96.472) -> (-18.288, 96.472) construction
  arc A9 (-13.51, 94.472) -> (-15.51, 96.472) centre (-15.51, 94.472) ccw construction
  line L19 (-13.51, 91.694) -> (-13.51, 94.472) construction
  line L20 (-13.51, 91.694) -> (-13.51, 43.354) construction
  arc A10 (-13.51, 43.354) -> (-11.51, 41.354) centre (-11.51, 43.354) ccw construction
  line L21 (-11.51, 41.354) -> (0.254, 41.354) construction
  line L22 (-11.51, 41.854) -> (0.254, 41.854)
  line L23 (2.524, 41.854) -> (0.254, 41.854)
  arc A11 (5.024, 39.354) -> (2.524, 41.854) centre (2.524, 39.354) ccw
  line L24 (5.024, 37.084) -> (5.024, 39.354)
  line L25 (5.024, 37.084) -> (5.024, 0)
  line L26 (5.024, 0) -> (5.024, -2.524)
  arc A12 (2.524, -5.024) -> (5.024, -2.524) centre (2.524, -2.524) ccw
  line L27 (0, -5.024) -> (2.524, -5.024)
  line L28 (-91.186, -5.024) -> (0, -5.024)
  line L29 (-91.186, -5.024) -> (-93.964, -5.024)
  arc A13 (-96.464, -2.524) -> (-93.964, -5.024) centre (-93.964, -2.524) ccw
  line L30 (-96.464, -2.524) -> (-96.464, 0.254)
  line L31 (-96.464, 91.948) -> (-96.464, 0.254)
  line L32 (-96.464, 94.472) -> (-96.464, 91.948)
  arc A14 (-93.964, 96.972) -> (-96.464, 94.472) centre (-93.964, 94.472) ccw
  line L33 (-91.44, 96.972) -> (-93.964, 96.972)
  line L34 (-18.288, 96.972) -> (-91.44, 96.972)
  line L35 (-15.51, 96.972) -> (-18.288, 96.972)
  arc A15 (-13.01, 94.472) -> (-15.51, 96.972) centre (-15.51, 94.472) ccw
  line L36 (-13.01, 91.694) -> (-13.01, 94.472)
  line L37 (-13.01, 91.694) -> (-13.01, 43.354)
  arc A16 (-13.01, 43.354) -> (-11.51, 41.854) centre (-11.51, 43.354) ccw
  dimension "d63" = -0.5
extrude "Extrude2'" cut sketch "Sketch2" against normal blind 2 bodies 2 in component "Case"
sketch "Sketch3 (2)" plane through (0, 0, 0) normal (0, 1, 0) x (1, 0, 0) in component "Case"
  line L0 (16.51, -91.694) -> (16.51, -39.624) construction
  arc A0 (16.51, -91.694) -> (18.288, -93.472) centre (18.288, -91.694) ccw construction
  line L1 (18.288, -93.472) -> (91.44, -93.472) construction
  arc A1 (91.44, -93.472) -> (92.964, -91.948) centre (91.44, -91.948) ccw construction
  line L2 (92.964, -91.948) -> (92.964, -0.254) construction
  arc A2 (92.964, -0.254) -> (91.186, 1.524) centre (91.186, -0.254) ccw construction
  line L3 (91.186, 1.524) -> (0, 1.524) construction
  arc A3 (0, 1.524) -> (-1.524, 0) centre (0, 0) ccw construction
  line L4 (-1.524, -37.084) -> (-1.524, 0) construction
  arc A4 (-1.524, -37.084) -> (-0.254, -38.354) centre (-0.254, -37.084) ccw construction
  line L5 (15.24, -38.354) -> (-0.254, -38.354) construction
  arc A5 (16.51, -39.624) -> (15.24, -38.354) centre (15.24, -39.624) ccw construction
  arc A6 (-2.524, -37.084) -> (-0.254, -39.354) centre (-0.254, -37.084) ccw
  line L6 (15.24, -39.354) -> (-0.254, -39.354)
  arc A7 (15.51, -39.624) -> (15.24, -39.354) centre (15.24, -39.624) ccw
  line L7 (15.51, -91.694) -> (15.51, -39.624)
  arc A8 (15.51, -91.694) -> (18.288, -94.472) centre (18.288, -91.694) ccw
  line L8 (18.288, -94.472) -> (91.44, -94.472)
  arc A9 (91.44, -94.472) -> (93.964, -91.948) centre (91.44, -91.948) ccw
  line L9 (93.964, -91.948) -> (93.964, -0.254)
  arc A10 (93.964, -0.254) -> (91.186, 2.524) centre (91.186, -0.254) ccw
  line L10 (91.186, 2.524) -> (0, 2.524)
  arc A11 (0, 2.524) -> (-2.524, 0) centre (0, 0) ccw
  line L11 (-2.524, -37.084) -> (-2.524, 0)
  dimension "d66" = 1
extrude "Extrude3" cut sketch "Sketch3 (2)" against normal blind 12 bodies 2 in component "Case"
move_body "Move1" bodies 2 to x (1, 0, 0) y (0, 1, 0) z (0, 0, 1) at (0, 2, 0) in component "Case"
sketch "Sketch4 (2)" plane through (0, -10, 0) normal (0, 1, 0) x (-1, 0, 0) in component "Case"
  arc A0 (-15.51, 91.694) -> (-18.288, 94.472) centre (-18.288, 91.694) ccw
  line L0 (-18.288, 94.472) -> (-91.44, 94.472)
  arc A1 (-91.44, 94.472) -> (-93.964, 91.948) centre (-91.44, 91.948) ccw
  line L1 (-93.964, 91.948) -> (-93.964, 0.254)
  arc A2 (-93.964, 0.254) -> (-91.186, -2.524) centre (-91.186, 0.254) ccw
  line L2 (-91.186, -2.524) -> (0, -2.524)
  arc A3 (0, -2.524) -> (2.524, 0) centre (0, 0) ccw
  line L3 (2.524, 0) -> (2.524, 37.084)
  arc A4 (2.524, 37.084) -> (0.254, 39.354) centre (0.254, 37.084) ccw
  line L4 (0.254, 39.354) -> (-15.24, 39.354)
  arc A5 (-15.51, 39.624) -> (-15.24, 39.354) centre (-15.24, 39.624) ccw
  line L5 (-15.51, 39.624) -> (-15.51, 91.694)
  circle A6 centre (-35.941, 9.906) radius 3.2553
  circle A7 centre (-89.408, 17.399) radius 3.2453
  circle A8 centre (-54.991, 55.499) radius 3.2528
  circle A9 centre (-89.408, 55.499) radius 3.2379
  circle A10 centre (-20.066, 74.613) radius 3.2553
  line L6 (-89.408, 20.6443) -> (-93.964, 20.6443)
  line L7 (-93.964, 20.6443) -> (-93.964, 14.1537)
  line L8 (-93.964, 14.1537) -> (-89.408, 14.1537)
  line L9 (-89.408, 14.1537) -> (-89.408, 20.6443)
  line L10 (-89.408, 58.7369) -> (-93.964, 58.7369)
  line L11 (-93.964, 58.7369) -> (-93.964, 52.2611)
  line L12 (-93.964, 52.2611) -> (-89.408, 52.2611)
  line L13 (-89.408, 52.2611) -> (-89.408, 58.7369)
  line L14 (-20.066, 77.8683) -> (-15.51, 77.8683)
  line L15 (-15.51, 77.8683) -> (-15.51, 71.3577)
  line L16 (-15.51, 71.3577) -> (-20.066, 71.3577)
  line L17 (-20.066, 71.3577) -> (-20.066, 77.8683)
  constraint horizontal L6
  constraint vertical L7
  constraint horizontal L8
  constraint vertical L9
  constraint coincident L1 L7.end
  constraint coincident A7 L6.start
  constraint horizontal L10
  constraint vertical L11
  constraint horizontal L12
  constraint vertical L13
  constraint coincident L1 L11.end
  constraint coincident A9 L10.start
  constraint tangent A9 L12
  constraint tangent A9 L10
  constraint tangent A7 L6
  constraint tangent A7 L8
  constraint horizontal L14
  constraint vertical L15
  constraint horizontal L16
  constraint vertical L17
  constraint coincident L5 L15.end
  constraint coincident A10 L14.start
  constraint tangent A10 L14
  constraint tangent A10 L16
extrude "Extrude4" add sketch "Sketch4 (2)" along normal blind 5 contours L5 A10 L14 L15 L16 | A10 L17 | A10 L17 | L1 A9 L10 L11 L12 | A9 L13 | A9 L13 | L1 A7 L6 L7 L8 | A7 L9 | A7 L9 | A6 | A8 bodies 2 in component "Case"
sketch "Sketch5" plane through (0, -5, 0) normal (0, 1, 0) x (-1, 0, 0) in component "Case"
  arc A0 (-20.066, 77.8683) -> (-20.066, 71.3577) centre (-20.066, 74.613) ccw
  line L0 (-20.066, 71.3577) -> (-15.51, 71.3577)
  line L1 (-15.51, 71.3577) -> (-15.51, 77.8683)
  line L2 (-15.51, 77.8683) -> (-20.066, 77.8683)
  circle A1 centre (-20.066, 74.613) radius 1.5875
  circle A2 centre (-35.941, 9.906) radius 1.5875
  circle A3 centre (-89.408, 17.399) radius 1.5875
  circle A4 centre (-89.408, 55.499) radius 1.5875
  circle A5 centre (-54.991, 55.499) radius 1.5875
  point P0 (-54.991, 55.499)
  point P1 (-89.408, 55.499)
  point P2 (-89.408, 17.399)
  point P3 (-35.941, 9.906)
  dimension "d71" = 3.175
  dimension "d72" = 3.175
  dimension "d73" = 3.175
  dimension "d74" = 3.175
  dimension "d75" = 3.175
  constraint concentric A0 A1
  constraint coincident P3 A2.centre
  constraint coincident P2 A3.centre
  constraint coincident P1 A4.centre
  constraint coincident P0 A5.centre
  measures "d71" diameter of A1
  measures "d72" diameter of A2
  measures "d73" diameter of A3
  measures "d74" diameter of A4
  measures "d75" diameter of A5
extrude "Extrude5" cut sketch "Sketch5" against normal blind 5 contours A1 | A2 | A3 | A4 | A5 bodies 2 in component "Case"